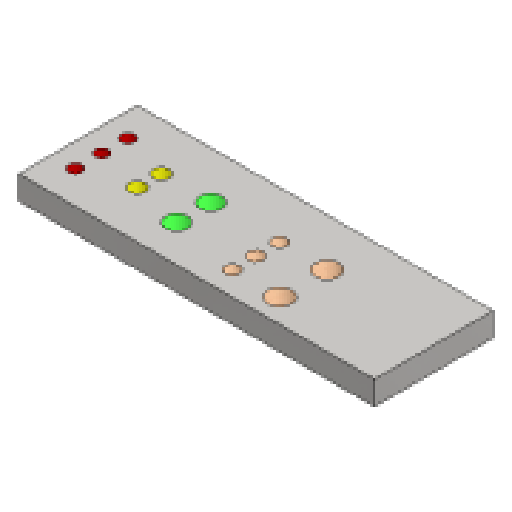
# Autodesk Inventor part: 홀간 거리 확인 파트-9
Saved by Autodesk Inventor 2026.1 (Build 301233000, 233)
## iProperties
Category: Title of a Parent object over this object
Company: Company
RuleStatus: InUse
Part Number: 홀간 거리 확인 파트-9
Project: Project Number
Checked By: Designed
Engr Approved By: Checked
User Status: ea / set
Material: SS400
Description: Description
Document SubType Name: Modeling
Mfg Approved By: Approved
Designer: suhyun-yoon
Stock Number: Stock Number
Density: 7.85 g/cm^3
Appearance: Plating Zinc White
Detail Description: Detail Description
Title: Title
Subject: Project Name
Author: suhyun-yoon
Revision Number: D
Autodesk Inventor part; units mm, degrees
ref_plane "YZ Plane" through (0, 0, 0) normal (1, 0, 0) x (0, 1, 0)
ref_plane "XZ Plane" through (0, 0, 0) normal (0, 1, 0) x (-1, 0, 0)
ref_plane "XY Plane" through (0, 0, 0) normal (0, 0, 1) x (1, 0, 0)
sketch "Sketch2" plane through (0, 0, 0) normal (0, 0, 1) x (1, 0, 0)
  line L0 (-75, -25) -> (75, -25)
  line L1 (75, -25) -> (75, 25)
  line L2 (75, 25) -> (-75, 25)
  line L3 (-75, 25) -> (-75, -25)
  line L4 (-75, -25) -> (75, 25) construction
  line L5 (75, -25) -> (-75, 25) construction
  point P0 (0, 0)
  dimension "d1" = 150
  dimension "d2" = 50
  constraints: 12 end point, 2 midpoint, 2 parallel, 1 horizontal, 1 perpendicular
  measures "d1" distance of L1.end L2.end
  measures "d2" distance of L2.end L0.start
extrude "Extrusion1" add sketch "Sketch2" along normal mid plane 10
sketch "Sketch3" plane through (0, 0, 5) normal (0, 0, 1) x (1, 0, 0)
  line L0 (-75, 25) -> (-75, -25) projected
  line L1 (75, 25) -> (-75, 25) projected
  point P0 (0, 0)
  point P1 (-65, 0)
  dimension "d40" = 10
  dimension "d43" = 25
  measures "d40" distance from line of L0 point (-65, 0)
  measures "d43" distance from line of L1 point (-65, 0)
hole "Hole1" at (-65, 0, 5) direction (0, 0, -1) diameter 5.5 depth 14.2 tip angle 118 clearance for "Socket Head Cap Screw" size "M5" standard "TS Profile"
sketch "Sketch4" plane through (0, 0, 5) normal (0, 0, 1) x (1, 0, 0)
  line L0 (-75, 25) -> (-75, -25) projected
  line L1 (75, 25) -> (-75, 25) projected
  point P0 (0, 0)
  point P1 (-45, 5)
  dimension "d41" = 30
  dimension "d42" = 20
  measures "d41" distance from line of L0 point (-45, 5)
  measures "d42" distance from line of point (-45, 5) L1
hole "Hole2" at (-45, 5, 5) direction (0, 0, -1) diameter 6.6 depth 14.2 tip angle 118 clearance for "Socket Head Cap Screw" size "M6" standard "TS Profile"
sketch "Sketch5" plane through (0, 0, 5) normal (0, 0, 1) x (1, 0, 0)
  line L0 (-75, 25) -> (-75, -25) projected
  line L1 (75, 25) -> (-75, 25) projected
  point P0 (0, 0)
  point P1 (-24, 5)
  dimension "d44" = 51
  dimension "d45" = 20
  measures "d44" distance from line of point (-24, 5) L0
  measures "d45" distance from line of L1 point (-24, 5)
hole "Hole3" at (-24, 5, 5) direction (0, 0, -1) diameter 9 depth 14.2 tip angle 118 clearance for "Socket Head Cap Screw" size "M8" standard "TS Profile"
sketch "Sketch6" plane through (0, 0, 5) normal (0, 0, 1) x (1, 0, 0)
  line L0 (-75, 25) -> (-75, -25) projected
  line L1 (75, 25) -> (-75, 25) projected
  point P0 (0, 0)
  point P1 (5, 5)
  dimension "d46" = 80
  dimension "d47" = 20
  measures "d46" distance from line of L0 point (5, 5)
  measures "d47" distance from line of L1 point (5, 5)
hole "Hole4" at (5, 5, 5) direction (0, 0, -1) diameter 6 depth 14.2 tip angle 118
sketch "Sketch7" plane through (0, 0, 5) normal (0, 0, 1) x (1, 0, 0)
  line L0 (-75, 25) -> (-75, -25) projected
  line L1 (75, 25) -> (-75, 25) projected
  point P0 (0, 0)
  point P1 (25, 5)
  dimension "d48" = 100
  dimension "d49" = 20
  measures "d48" distance from line of L0 point (25, 5)
  measures "d49" distance from line of L1 point (25, 5)
hole "Hole5" at (25, 5, 5) direction (0, 0, -1) diameter 10 depth 14.2 tip angle 118
pattern_linear "Rectangular Pattern1" count 3 spacing 11 along (0, -1, 0) of "Hole1" first direction both ways yes
pattern_linear "Rectangular Pattern2" count 2 spacing 10 along (0, -1, 0) of "Hole2"
pattern_linear "Rectangular Pattern3" count 2 spacing 14.5 along (0, -1, 0) of "Hole3"
pattern_linear "Rectangular Pattern4" count 3 spacing 10 along (0, -1, 0) of "Hole4"
pattern_linear "Rectangular Pattern5" count 2 spacing 20 along (0, -1, 0) of "Hole5"
body "Solid1"
